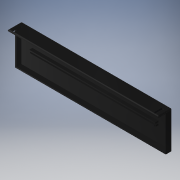
# Autodesk Inventor part: Basket
Saved by Autodesk Inventor 2019.3 (Build 233278000, 278)
## iProperties
Created: 2020-10-08
Part Number: Basket
Material: Acetalharz, Schwarz
Document SubType Name: Modeling
Designer: Nicolas Frick
Density: 1.425 g/cm^3
Appearance: Glatt - Schwarz
Author: Nicolas Frick
Autodesk Inventor part; units mm, degrees
ref_plane "YZ Plane" through (0, 0, 0) normal (1, 0, 0) x (0, 1, 0)
ref_plane "XZ Plane" through (0, 0, 0) normal (0, 1, 0) x (-1, 0, 0)
ref_plane "XY Plane" through (0, 0, 0) normal (0, 0, 1) x (1, 0, 0)
sketch "Skizze2" plane through (0, 0, 0) normal (0, 0, 1) x (1, 0, 0)
  line L0 (-122.5, 30) -> (122.5, 30)
  line L1 (122.5, 30) -> (122.5, -30)
  line L2 (122.5, -30) -> (-122.5, -30)
  line L3 (-122.5, -30) -> (-122.5, 30)
  line L4 (-122.5, 30) -> (122.5, -30) construction
  line L5 (122.5, 30) -> (-122.5, -30) construction
  point P0 (0, 0)
  dimension "d0" = 245
  dimension "d1" = 60
  constraints: 12 end point, 2 midpoint, 2 parallel, 1 horizontal, 1 perpendicular
  measures "d0" distance of L1.end L2.end
  measures "d1" distance of L0.end L1.end
extrude "Extrusion1" add sketch "Skizze2" along normal blind 2.5
sketch "Skizze3" plane through (0, 0, 2.5) normal (0, 0, 1) x (1, 0, 0)
  line L0 (122.5, 30) -> (-122.5, 30) construction
  line L1 (-122.5, 30) -> (-122.5, -30) construction
  line L2 (-122.5, -30) -> (122.5, -30) construction
  line L3 (122.5, -30) -> (122.5, 30) construction
  line L4 (122.5, 30) -> (-122.5, 30) projected
  line L5 (122.5, -30) -> (122.5, 30) projected
  line L6 (-122.5, 30) -> (122.5, 30)
  line L7 (122.5, 30) -> (122.5, 27.5)
  line L8 (122.5, 27.5) -> (-122.5, 27.5)
  line L9 (-122.5, 27.5) -> (-122.5, 30)
  point P0 (0, 0)
  dimension "d4" = 2.5
  constraints: 8 end point, 2 parallel, 1 horizontal, 1 perpendicular, 1 point on line
  measures "d4" distance of L6.end L7.end
extrude "Extrusion2" add sketch "Skizze3" along normal blind 20
sketch "Skizze4" plane through (-122.5, 30, 0) normal (0, 1, 0) x (1, 0, 0)
  line L0 (0, 0) -> (245, 0) construction
  line L1 (0, 0) -> (0, -22.5) construction
  line L2 (245, -22.5) -> (0, -22.5) construction
  line L3 (245, 0) -> (245, -22.5) construction
  line L4 (122.5, 0) -> (7, 0) construction
  line L5 (0, 0) -> (245, 0) construction
  line L6 (7, 0) -> (238, 0) construction
  line L7 (7, -22.5) -> (7, -14.5) construction
  line L8 (245, -22.5) -> (0, -22.5) projected
  line L9 (238, -22.5) -> (238, -14.5) construction
  line L10 (7, -19.5) -> (7, -9.5) construction
  line L11 (9, -19.5) -> (9, -9.5)
  line L12 (5, -9.5) -> (5, -19.5)
  arc A0 (5, -19.5) -> (9, -19.5) centre (7, -19.5) ccw
  arc A1 (9, -9.5) -> (5, -9.5) centre (7, -9.5) ccw
  line L13 (238, -9.5) -> (238, -19.5) construction
  line L14 (236, -9.5) -> (236, -19.5)
  line L15 (240, -19.5) -> (240, -9.5)
  arc A2 (240, -9.5) -> (236, -9.5) centre (238, -9.5) ccw
  arc A3 (236, -19.5) -> (240, -19.5) centre (238, -19.5) ccw
  dimension "d8" = 231
  dimension "d9" = 8
  dimension "d10" = 5
  dimension "d11" = 4
  dimension "d12" = 8
  dimension "d13" = 5
  dimension "d14" = 4
  constraints: 24 end point, 8 point on circle, 8 tangent, 5 point on line, 4 centre point, 2 midpoint, 2 parallel, 2 vertical, 1 perpendicular
  measures "d8" distance of L4.end L6.end
  measures "d9" distance of L7.start L7.end
  measures "d10" distance of L7.end L10.end
  measures "d11" diameter of A1
  measures "d12" distance of L9.end L9.start
  measures "d13" distance of L9.end L13.end
  measures "d14" diameter of A3
extrude "Extrusion3" cut sketch "Skizze4" against normal blind 20
sketch "Skizze5" plane through (0, 0, 2.5) normal (0, 0, 1) x (1, 0, 0)
  line L0 (122.5, 27.5) -> (-122.5, 27.5) construction
  line L1 (-122.5, 27.5) -> (-122.5, -30) construction
  line L2 (-122.5, -30) -> (122.5, -30) construction
  line L3 (122.5, -30) -> (122.5, 27.5) construction
  line L4 (122.5, -30) -> (122.5, 27.5) projected
  line L5 (122.5, 27.5) -> (122.5, -30)
  line L6 (122.5, -30) -> (-122.5, -30)
  line L7 (-122.5, -30) -> (-122.5, 27.5)
  line L8 (-122.5, 24.8143) -> (-120.5, 24.8143) construction
  line L9 (122.5, 16.3856) -> (120.5, 16.3856) construction
  line L10 (-122.5, -30) -> (122.5, -30) projected
  line L11 (0, -30) -> (0, -28) construction
  line L12 (120.5, 27.5) -> (120.5, -28)
  line L13 (120.5, -28) -> (-120.5, -28)
  line L14 (-120.5, -28) -> (-120.5, 27.5)
  line L15 (-122.5, 27.5) -> (-120.5, 27.5)
  line L16 (120.5, 27.5) -> (122.5, 27.5)
  point P0 (0, 0)
  dimension "d17" = 2
  dimension "d18" = 2
  dimension "d19" = 2
  constraints: 22 end point, 4 parallel, 4 perpendicular, 2 horizontal, 2 point on line, 1 midpoint, 1 vertical
  measures "d17" distance of L8.start L8.end
  measures "d18" distance of L9.start L9.end
  measures "d19" distance of L11.start L11.end
extrude "Extrusion4" add sketch "Skizze5" along normal blind 8
fillet "Rundung1" radius 2 7 edges at (-122.5, 30, 11.25) (0, 30, 0) (122.5, 30, 11.25) (0, 30, 22.5) (122.5, 0, 0) (-122.5, 0, 0) (0, -30, 0)
sketch "Skizze7" plane through (0, 0, 0) normal (0, 0, -1) x (-1, 0, 0)
  line L0 (120.5, 30) -> (-120.5, 30) construction
  line L1 (122.5, -30) -> (122.5, 28) construction
  line L2 (-122.5, -30) -> (122.5, -30) construction
  line L3 (-122.5, 28) -> (-122.5, -30) construction
  line L4 (0, 30) -> (0, 0) construction
  line L5 (-102.5, 0.65) -> (102.5, 0.65)
  line L6 (102.5, 0.65) -> (102.5, -0.65)
  line L7 (102.5, -0.65) -> (-102.5, -0.65)
  line L8 (-102.5, -0.65) -> (-102.5, 0.65)
  line L9 (-102.5, 0.65) -> (102.5, -0.65) construction
  line L10 (102.5, 0.65) -> (-102.5, -0.65) construction
  dimension "d28" = 205
  dimension "d29" = 1.3
  constraints: 14 end point, 3 midpoint, 2 parallel, 1 horizontal, 1 perpendicular, 1 vertical
  measures "d28" distance of L6.end L7.end
  measures "d29" distance of L5.end L6.end
extrude "Extrusion6" cut sketch "Skizze7" against normal blind 5
sketch "Skizze8" plane through (0, 0, 2.5) normal (0, 0, 1) x (1, 0, 0)
  line L0 (102.5, -0.65) -> (-102.5, -0.65) construction
  line L1 (-102.5, -0.65) -> (102.5, -0.65)
  line L2 (102.5, -0.65) -> (102.5, -2.6532)
  line L3 (102.5, -2.6532) -> (-102.5, -2.6532)
  line L4 (-102.5, -2.6532) -> (-102.5, -0.65)
  point P0 (0, 0)
  constraints: 8 end point, 2 parallel, 1 horizontal, 1 perpendicular
extrude "Extrusion7" add sketch "Skizze8" along normal blind 5
fillet "Rundung2" radius 2 2 edges at (-102.5, -1.6516, 7.5) (102.5, -1.6516, 7.5)
sketch "Skizze9" plane through (0, 0, 2.5) normal (0, 0, 1) x (1, 0, 0)
  line L0 (-102.5, 0.65) -> (102.5, 0.65) construction
  line L1 (100.5, -0.65) -> (-100.5, -0.65) construction
  line L2 (-102.5, 0.65) -> (102.5, 0.65)
  line L3 (102.5, 0.65) -> (102.5, 1.65)
  line L4 (102.5, 1.65) -> (-102.5, 1.65)
  line L5 (-102.5, 1.65) -> (-102.5, 0.65)
  point P0 (0, 0)
  dimension "d35" = 1
  constraints: 8 end point, 2 parallel, 1 horizontal, 1 perpendicular
  measures "d35" distance of L3.end L2.end
extrude "Extrusion8" cut sketch "Skizze9" against normal blind 10
sketch "Skizze10" plane through (0, 0, 2.5) normal (0, 0, 1) x (1, 0, 0)
  line L0 (-102.5, 1.65) -> (102.5, 1.65) projected
  line L1 (-102.5, 1.65) -> (102.5, 1.65)
  line L2 (102.5, 1.65) -> (102.5, 3.65)
  line L3 (102.5, 3.65) -> (-102.5, 3.65)
  line L4 (-102.5, 3.65) -> (-102.5, 1.65)
  point P0 (0, 0)
  dimension "d38" = 2
  constraints: 8 end point, 2 parallel, 1 horizontal, 1 perpendicular
  measures "d38" distance of L2.end L1.end
extrude "Extrusion9" add sketch "Skizze10" along normal blind 5
